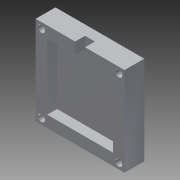
# Autodesk Inventor part: NEMA_17-back
Saved by Autodesk Inventor 2013 (Build 170138000, 138)
## iProperties
Created: 2013-09-16
Part Number: NEMA_17-back
Material: Aluminum 6061
Document SubType Name: Modeling
Designer: Ian
Density: 1 g/cm^3
Author: Ian
Autodesk Inventor part; units mm, degrees
ref_plane "YZ Plane" through (0, 0, 0) normal (1, 0, 0) x (0, 1, 0)
ref_plane "XZ Plane" through (0, 0, 0) normal (0, 1, 0) x (-1, 0, 0)
ref_plane "XY Plane" through (0, 0, 0) normal (0, 0, 1) x (1, 0, 0)
sketch "Sketch1" plane through (0, 0, 0) normal (0, 0, 1) x (1, 0, 0)
  line L0 (-28.575, -28.575) -> (28.575, -28.575)
  line L1 (28.575, -28.575) -> (28.575, 28.575)
  line L2 (28.575, 28.575) -> (-28.575, 28.575)
  line L3 (-28.575, 28.575) -> (-28.575, -28.575)
  line L4 (-28.575, -28.575) -> (28.575, 28.575) construction
  line L5 (28.575, -28.575) -> (-28.575, 28.575) construction
  point P0 (0, 0)
  dimension "d0" = 57.15
  dimension "d1" = 57.15
  constraints: 12 end point, 2 midpoint, 2 parallel, 1 horizontal, 1 perpendicular
  measures "d0" distance of L2.end L1.end
  measures "d1" distance of L1.end L0.end
extrude "Extrusion1" add sketch "Sketch1" along normal blind 12.7
sketch "Sketch2" plane through (0, 0, 12.7) normal (0, 0, 1) x (1, 0, 0)
  line L0 (-21.15, -21.15) -> (21.15, -21.15)
  line L1 (21.15, -21.15) -> (21.15, 21.15)
  line L2 (21.15, 21.15) -> (-21.15, 21.15)
  line L3 (-21.15, 21.15) -> (-21.15, -21.15)
  line L4 (-21.15, -21.15) -> (21.15, 21.15) construction
  line L5 (21.15, -21.15) -> (-21.15, 21.15) construction
  point P0 (0, 0)
  dimension "d4" = 42.3
  dimension "d5" = 42.3
  constraints: 12 end point, 2 midpoint, 2 parallel, 1 horizontal, 1 perpendicular
  measures "d4" distance of L2.end L1.end
  measures "d5" distance of L1.end L0.end
extrude "Extrusion2" cut sketch "Sketch2" against normal blind 6.35
sketch "Sketch3" plane through (-21.15, 21.15, 12.7) normal (0, -1, 0) x (1, 0, 0)
  line L0 (0, 0) -> (42.3, 0) projected
  line L1 (0, 0) -> (0, -6.35) projected
  line L2 (0, -6.35) -> (42.3, -6.35) projected
  line L3 (42.3, 0) -> (42.3, -6.35) projected
  line L4 (21.15, -6.35) -> (24.325, -6.35)
  line L5 (24.325, -6.35) -> (24.325, 0)
  line L6 (24.325, 0) -> (21.15, 0)
  line L7 (21.15, -6.35) -> (17.975, -6.35)
  line L8 (17.975, -6.35) -> (17.975, 0)
  line L9 (17.975, 0) -> (21.15, 0)
  point P0 (21.15, -12.7)
  dimension "d10" = 17.975
  dimension "d11" = 17.975
  constraints: 12 end point, 2 horizontal, 2 parallel, 2 perpendicular, 2 point on line, 1 midpoint
  measures "d10" distance between parallel lines of L1 L8
  measures "d11" distance between parallel lines of L3 L5
extrude "Extrusion3" cut sketch "Sketch3" against normal up to next contours L0 L5 L2 L8
sketch "Sketch4" plane through (0, 0, 12.7) normal (0, 0, 1) x (1, 0, 0)
  line L0 (28.575, -28.575) -> (28.575, 28.575) projected
  line L1 (28.575, 28.575) -> (3.175, 28.575) projected
  line L2 (28.575, 28.575) -> (-28.575, -28.575) construction
  line L3 (-28.575, 28.575) -> (28.575, -28.575) construction
  line L4 (28.575, 24.8625) -> (24.8625, 24.8625) construction
  line L5 (-24.8625, -24.8625) -> (24.8625, -24.8625) construction
  line L6 (24.8625, -24.8625) -> (24.8625, 24.8625) construction
  line L7 (24.8625, 24.8625) -> (-24.8625, 24.8625) construction
  line L8 (-24.8625, 24.8625) -> (-24.8625, -24.8625) construction
  line L9 (-24.8625, -24.8625) -> (24.8625, 24.8625) construction
  line L10 (24.8625, -24.8625) -> (-24.8625, 24.8625) construction
  point P0 (0, 0)
  dimension "d14" = 3.7125
  constraints: 18 end point, 4 coincident, 3 parallel, 3 point on line, 2 midpoint, 2 perpendicular, 1 horizontal
  measures "d14" distance between parallel lines of L1 L7
hole "Hole1" at (-24.8625, 24.8625, 12.7) at (24.8625, 24.8625, 12.7) at (24.8625, -24.8625, 12.7) at (-24.8625, -24.8625, 12.7) direction (0, 0, -1) diameter 4.4958 end through all clearance for "Flat Head Machine Screw (82)" size "#8" standard "Ansi Unified Screw Threads"
sketch "Sketch5" plane through (-28.575, -28.575, 0) normal (0, -1, 0) x (1, 0, 0)
  line L0 (57.15, 0) -> (57.15, 12.7) projected
  line L1 (0, 12.7) -> (57.15, 12.7) projected
  line L2 (0, 0) -> (0, 12.7) projected
  line L3 (3.9568, 4.7625) -> (48.9174, 4.7625) construction
  point P0 (28.575, 0)
  point P1 (10.16, 4.7625)
  point P2 (46.99, 4.7625)
  dimension "d22" = 7.9375
  dimension "d23" = 10.16
  dimension "d24" = 10.16
  constraints: 2 end point, 2 point on line, 1 perpendicular
  measures "d22" distance between parallel lines of L1 L3
  measures "d23" distance from line of L2 point (10.16, 4.762)
  measures "d24" distance from line of L0 point (46.99, 4.763)
hole "Hole2" at (-18.415, -28.575, 4.7625) at (18.415, -28.575, 4.7625) direction (0, 1, 0) diameter 4.3434 depth 6.35 tip angle 118 thread size "12-24 UNC" class "2B" standard "ANSI Unified Screw Threads"
equation "\"d1\" = d0"
equation "\"d11\" = d10"
equation "\"d24\" = d23"
body "Solid1"
